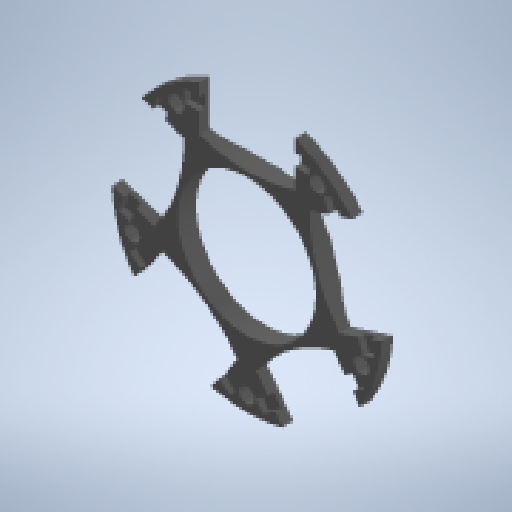
# Autodesk Inventor part: wheel_body_front_outside
Saved by Autodesk Inventor 2024.1 (Build 281209000, 209)
## iProperties
Created: 2024-11-26
Part Number: wheel_body_front_outside
Material: 一般
Document SubType Name: Modeling
Designer: hibik
Density: 1 g/cm^3
Appearance: 既定
Author: hibik
Autodesk Inventor part; units mm, degrees
ref_plane "YZ Plane" through (0, 0, 0) normal (1, 0, 0) x (0, 1, 0)
ref_plane "XZ Plane" through (0, 0, 0) normal (0, 1, 0) x (-1, 0, 0)
ref_plane "XY Plane" through (0, 0, 0) normal (0, 0, 1) x (1, 0, 0)
sketch "スケッチ1" plane through (0, 0, 0) normal (0, 0, 1) x (1, 0, 0)
  arc A0 (-9.75, 17.6881) -> (9.75, 17.6881) centre (0, 45) ccw
  arc A1 (-9.75, 16.6286) -> (9.75, 16.6286) centre (0, 45) ccw
  line L0 (-9.75, 42) -> (9.75, 42)
  line L1 (9.75, 42) -> (9.75, 15)
  line L2 (9.75, 15) -> (-9.75, 15)
  line L3 (-9.75, 15) -> (-9.75, 42)
  line L4 (-9.75, 29) -> (9.75, 29)
  circle A2 centre (0, 0) radius 14
  circle A3 centre (0, 0) radius 15 construction
  circle A4 centre (0, 0) radius 29
  line L5 (-17.2788, -4.6375) -> (-42.9573, 3.7059)
  arc A5 (-18.8276, -4.1343) -> (-12.8018, 14.4113) centre (-42.7975, 13.9058) ccw
  line L6 (-36.9315, 22.2515) -> (-11.2529, 13.9081)
  line L7 (-0.9289, -17.8662) -> (-16.7991, -39.7096)
  arc A6 (-1.8861, -19.1837) -> (-17.6619, -7.7219) centre (-26.4503, -36.4058) ccw
  line L8 (-32.5749, -28.2478) -> (-16.7047, -6.4043)
  line L9 (16.7047, -6.4043) -> (32.5749, -28.2478)
  arc A7 (17.6619, -7.7219) -> (1.8861, -19.1837) centre (26.4503, -36.4058) ccw
  line L10 (16.7991, -39.7096) -> (0.9289, -17.8662)
  line L11 (11.2529, 13.9081) -> (36.9315, 22.2515)
  arc A8 (12.8018, 14.4113) -> (18.8276, -4.1343) centre (42.7975, 13.9058) ccw
  line L12 (42.9573, 3.7059) -> (17.2788, -4.6375)
  circle A9 centre (0, 0) radius 27.5
  line L13 (-9.75, 16.6286) -> (-9.75, 27.3119)
  point P0 (0, 42)
  point P1 (-19.8353, -3.8069)
  point P2 (-24.5677, 18.2343)
  point P3 (-13.8095, 14.7387)
  point P4 (-2.5089, -20.0409)
  point P5 (-24.9337, -17.7306)
  point P6 (-18.2847, -8.5791)
  point P7 (18.2847, -8.5791)
  point P8 (9.1579, -29.1924)
  point P9 (2.5089, -20.0409)
  point P10 (13.8095, 14.7387)
  point P11 (30.5936, -0.3113)
  point P12 (19.8353, -3.8069)
  point P13 (9.75, 25.7136)
  point P14 (-9.75, 25.7136)
  point P15 (-21.4421, 17.2187)
  point P16 (-27.468, -1.3269)
  point P17 (-23.002, -15.0718)
  point P18 (-7.2261, -26.5336)
  point P19 (7.2261, -26.5336)
  point P20 (23.002, -15.0718)
  point P21 (27.468, -1.3269)
  point P22 (21.4421, 17.2187)
  point P23 (0, 15)
  point P24 (-9.75, 21.9702)
  dimension "d110" = 58
  dimension "d2" = 14
  dimension "d3" = 13
  dimension "d4" = 19.5
  dimension "d9" = 29
  dimension "d10" = 1
  dimension "d16" = 360
  dimension "d18" = 1.5
  dimension "d108" = 14
  dimension "d122" = 1
  constraints: 28 end point, 26 point on line, 12 point on circle, 9 centre point, 6 coincident, 2 horizontal, 2 midpoint, 2 parallel, 2 perpendicular, 2 tangent, 2 vertical alignment, 69 other
  measures "d2" distance between parallel lines of L2 L4
  measures "d3" distance between parallel lines of L0 L4
  measures "d4" distance of L0.start L0.end
  measures "d9" radius of A0
  measures "d10" radial gap between concentric circles of A0 A1
  measures "d122" radial gap between concentric circles of A3 A2
extrude "押し出し1" add sketch "スケッチ1" along normal blind 3.75 contours L3 L2 L1 A9 L11 A8 L12 L9 A7 L10 L7 A6 L8 L5 A5 L6 | A1 L2 L3 | L1 L2 A1
sketch "スケッチ2" plane through (0, 0, 3.75) normal (0, 0, 1) x (1, 0, 0)
  line L0 (-13.4426, 18.5021) -> (0, 0) construction
  line L1 (-9.75, 16.6286) -> (-9.75, 25.7136) projected
  line L2 (-21.4421, 17.2187) -> (-12.8018, 14.4113) projected
  arc A0 (-9.75, 25.7136) -> (-21.4421, 17.2187) centre (0, 0) ccw projected
  circle A1 centre (-14.4007, 19.8209) radius 1.6
  line L3 (-14.4007, 19.8209) -> (-16.7444, 18.1181)
  circle A2 centre (0, 0) radius 14 projected
  circle A3 centre (0, 0) radius 24.5 construction
  circle A4 centre (-23.3009, -7.5709) radius 1.6
  circle A5 centre (0, -24.5) radius 1.6
  circle A6 centre (23.3009, -7.5709) radius 1.6
  circle A7 centre (14.4007, 19.8209) radius 1.6
  point P0 (-9.75, 57.7)
  point P1 (9.75, 25.7136)
  point P2 (-9.75, 17.6881)
  dimension "d22" = 36
  dimension "d23" = 36
  dimension "d34" = 28
  dimension "d111" = 3.2
  dimension "d113" = 3
  dimension "d116" = 360
  constraints: 5 centre point, 4 end point, 1 coincident, 1 line through centre, 1 perpendicular, 1 point on line, 14 other
  measures "d22" angle of L1 L0
  measures "d23" angle of L2 L0
  measures "d34" diameter of A2
  measures "d111" diameter of A1
extrude "押し出し2" cut sketch "スケッチ2" against normal through all contours A1 | A4 | A5 | A6 | A7
sketch "スケッチ3" plane through (0, 0, 3.75) normal (0, 0, 1) x (1, 0, 0)
  line L0 (-9.75, 20.6803) -> (-12.75, 20.6803)
  line L1 (-12.75, 20.6803) -> (-12.75, 23.1803)
  line L2 (-12.75, 23.1803) -> (-9.75, 23.1803)
  line L3 (-9.75, 23.1803) -> (-9.75, 20.6803)
  line L4 (9.75, 20.6803) -> (12.75, 20.6803)
  line L5 (12.75, 20.6803) -> (12.75, 23.1803)
  line L6 (12.75, 23.1803) -> (9.75, 23.1803)
  line L7 (9.75, 23.1803) -> (9.75, 20.6803)
  line L8 (-22.681, -2.8822) -> (-23.6081, -5.7354)
  line L9 (-23.6081, -5.7354) -> (-25.9857, -4.9629)
  line L10 (-25.9857, -4.9629) -> (-25.0587, -2.1097)
  line L11 (-25.0587, -2.1097) -> (-22.681, -2.8822)
  line L12 (-19.0328, 16.4359) -> (-16.6552, 15.6634)
  line L13 (-16.6552, 15.6634) -> (-15.7282, 18.5165)
  line L14 (-15.7282, 18.5165) -> (-18.1058, 19.2891)
  line L15 (-18.1058, 19.2891) -> (-19.0328, 16.4359)
  line L16 (-4.2677, -22.4616) -> (-1.8406, -24.225)
  line L17 (-1.8406, -24.225) -> (-3.3101, -26.2475)
  line L18 (-3.3101, -26.2475) -> (-5.7371, -24.4842)
  line L19 (-5.7371, -24.4842) -> (-4.2677, -22.4616)
  line L20 (-21.5129, -13.0223) -> (-20.0435, -10.9998)
  line L21 (-20.0435, -10.9998) -> (-22.4705, -9.2364)
  line L22 (-22.4705, -9.2364) -> (-23.94, -11.259)
  line L23 (-23.94, -11.259) -> (-21.5129, -13.0223)
  line L24 (20.0435, -10.9998) -> (22.4705, -9.2364)
  line L25 (22.4705, -9.2364) -> (23.94, -11.259)
  line L26 (23.94, -11.259) -> (21.5129, -13.0223)
  line L27 (21.5129, -13.0223) -> (20.0435, -10.9998)
  line L28 (5.7371, -24.4842) -> (4.2677, -22.4616)
  line L29 (4.2677, -22.4616) -> (1.8406, -24.225)
  line L30 (1.8406, -24.225) -> (3.3101, -26.2475)
  line L31 (3.3101, -26.2475) -> (5.7371, -24.4842)
  line L32 (16.6552, 15.6634) -> (15.7282, 18.5165)
  line L33 (15.7282, 18.5165) -> (18.1058, 19.2891)
  line L34 (18.1058, 19.2891) -> (19.0328, 16.4359)
  line L35 (19.0328, 16.4359) -> (16.6552, 15.6634)
  line L36 (25.0587, -2.1097) -> (22.681, -2.8822)
  line L37 (22.681, -2.8822) -> (23.6081, -5.7354)
  line L38 (23.6081, -5.7354) -> (25.9857, -4.9629)
  line L39 (25.9857, -4.9629) -> (25.0587, -2.1097)
  line L40 (-9.75, 16.6286) -> (-9.75, 25.7136) projected
  line L41 (9.75, 25.7136) -> (9.75, 16.6286) projected
  arc A0 (-12.8007, 19.8209) -> (-12.8007, 19.8209) centre (-14.4007, 19.8209) ccw projected
  circle A1 centre (0, 0) radius 24
  circle A2 centre (0, 0) radius 14 projected
  point P0 (-9.75, 21.9303)
  point P1 (-23.8699, -2.496)
  point P2 (-5.0024, -23.4729)
  point P3 (20.7782, -12.0111)
  point P4 (17.844, 16.0496)
  point P5 (-9.75, 17.6881)
  point P6 (9.75, 17.6881)
  point P7 (9.75, 21.9303)
  dimension "d40" = 2.5
  dimension "d45" = 360
  dimension "d105" = 3
  dimension "d107" = 10
  constraints: 80 end point, 10 point on line, 4 parallel, 3 collinear, 2 horizontal, 2 midpoint, 2 perpendicular, 1 coincident, 1 horizontal alignment, 89 other
  measures "d40" distance of L0.end L1.end
  measures "d105" distance of L1.end L2.end
extrude "押し出し3" cut sketch "スケッチ3" against normal blind 1.25 contours L0 A1 L3 | L0 L1 L2 L3 A1 | A1 L4 L7 | L7 L6 L5 L4 A1 | A1 L12 L15 L14 L13 | L13 L12 A1 | A1 L35 L32 | L32 L33 L34 L35 A1 | A1 L8 L9 L10 L11 | L11 L8 A1 | A1 L37 L36 | L36 L39 L38 L37 A1 | A1 L20 L23 L22 L21 | L21 L20 A1 | A1 L27 L24 | L24 L25 L26 L27 A1 | A1 L16 L17 L18 L19 | L19 L16 A1 | A1 L29 L28 | L28 L31 L30 L29 A1
sketch "スケッチ15" plane through (0, 0, 0) normal (0, 0, -1) x (-1, 0, 0)
  circle A0 centre (0, 0) radius 15.5
  arc A1 (-9.75, 16.6286) -> (9.75, 16.6286) centre (0, 45) ccw projected
  circle A2 centre (-23.3009, -7.5709) radius 1.6 projected
  circle A3 centre (-14.4007, 19.8209) radius 1.6 projected
  circle A4 centre (0, -24.5) radius 1.6 projected
  circle A5 centre (14.4007, 19.8209) radius 1.6 projected
  circle A6 centre (23.3009, -7.5709) radius 1.6 projected
  line L0 (-27.468, -1.3269) -> (-18.8276, -4.1343) projected
  arc A7 (-27.468, -1.3269) -> (-23.002, -15.0718) centre (0, 0) ccw projected
  line L1 (-17.6619, -7.7219) -> (-23.002, -15.0718) projected
  arc A8 (-1.8861, -19.1837) -> (-17.6619, -7.7219) centre (-26.4503, -36.4058) ccw projected
  line L2 (-7.2261, -26.5336) -> (-1.8861, -19.1837) projected
  arc A9 (-7.2261, -26.5336) -> (7.2261, -26.5336) centre (0, 0) ccw projected
  line L3 (1.8861, -19.1837) -> (7.2261, -26.5336) projected
  arc A10 (17.6619, -7.7219) -> (1.8861, -19.1837) centre (26.4503, -36.4058) ccw projected
  line L4 (23.002, -15.0718) -> (17.6619, -7.7219) projected
  arc A11 (23.002, -15.0718) -> (27.468, -1.3269) centre (0, 0) ccw projected
  line L5 (18.8276, -4.1343) -> (27.468, -1.3269) projected
  arc A12 (12.8018, 14.4113) -> (18.8276, -4.1343) centre (42.7975, 13.9058) ccw projected
  line L6 (21.4421, 17.2187) -> (12.8018, 14.4113) projected
  arc A13 (21.4421, 17.2187) -> (9.75, 25.7136) centre (0, 0) ccw projected
  line L7 (9.75, 16.6286) -> (9.75, 25.7136) projected
  arc A14 (-9.75, 16.6286) -> (9.75, 16.6286) centre (0, 45) ccw projected
  line L8 (-9.75, 25.7136) -> (-9.75, 16.6286) projected
  arc A15 (-9.75, 25.7136) -> (-21.4421, 17.2187) centre (0, 0) ccw projected
  line L9 (-12.8018, 14.4113) -> (-21.4421, 17.2187) projected
  arc A16 (-18.8276, -4.1343) -> (-12.8018, 14.4113) centre (-42.7975, 13.9058) ccw projected
  circle A17 centre (0, 0) radius 14 projected
  circle A18 centre (0, 0) radius 15 construction
  point P0 (11.4923, -10.4008)
  point P1 (-6.3405, -14.1439)
  point P2 (13.4431, 7.7158)
  point P3 (9.75, 16.6286)
  point P4 (3.184, 15.1694)
  point P5 (-9.75, 16.6286)
  point P6 (-15.4109, 1.6594)
  point P7 (6.3405, -14.1439)
  point P8 (15.4109, 1.6594)
  point P9 (3.184, 15.1694)
  point P10 (-13.4431, 7.7158)
  point P11 (-3.184, 15.1694)
  point P12 (-11.4923, -10.4008)
  dimension "d125" = 0.5
  constraints: 2 centre point, 2 coincident, 1 tangent
  measures "d125" radial gap between concentric circles of A0 A18
extrude "押し出し15" cut sketch "スケッチ15" against normal blind 1.5 contours A0 A12 L5 A11 L4 A10 | A0 A10 | A0 A1 L7 A13 L6 A12 | A10 L3 A9 L2 A8 A0 | A0 A8 | A0 A16 L9 A15 L8 A1 | A8 L1 A7 L0 A16 A0 | A16 A0
fillet "フィレット9" radius 7 5 edges at (9.1107, 12.5398, 1.5) (-9.1107, 12.5398, 1.5) (-14.7414, -4.7898, 1.5) (0, -15.5, 1.5) (14.7414, -4.7898, 1.5)
equation "\"d22\" = d23"
